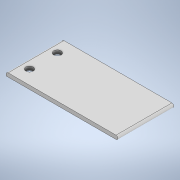
# Autodesk Inventor part: Cover
Saved by Autodesk Inventor 2020 (Build 240168000, 168)
## iProperties
Created: 2020-02-19
Part Number: Cover
Material: Generic
Document SubType Name: Modeling
Designer: maple
Density: 1 g/cm^3
Appearance: Default
Author: maple
Autodesk Inventor part; units mm, degrees
ref_plane "YZ Plane" through (0, 0, 0) normal (1, 0, 0) x (0, 1, 0)
ref_plane "XZ Plane" through (0, 0, 0) normal (0, 1, 0) x (-1, 0, 0)
ref_plane "XY Plane" through (0, 0, 0) normal (0, 0, 1) x (1, 0, 0)
sketch "Sketch1" plane through (0, 0, 0) normal (0, 1, 0) x (-1, 0, 0)
  line L0 (0, 0) -> (-76.2, 0)
  line L1 (-76.2, 0) -> (-76.2, -38.1)
  line L2 (-76.2, -38.1) -> (0, -38.1)
  line L3 (0, -38.1) -> (0, 0)
  dimension "d0" = 76.2
  dimension "d1" = 38.1
  constraints: 8 end point, 2 parallel, 1 horizontal, 1 perpendicular
  measures "d0" distance of L2.end L1.end
  measures "d1" distance of L1.end L0.end
extrude "Extrusion1" add sketch "Sketch1" along normal blind 2.54
sketch "Sketch2" plane through (0, 2.54, 0) normal (0, 1, 0) x (1, 0, 0)
  line L0 (0, 0) -> (6.35, 0)
  line L1 (0, 0) -> (76.2, 0) projected
  line L2 (6.35, 0) -> (6.35, 38.1)
  line L3 (76.2, 38.1) -> (0, 38.1) projected
  line L4 (6.35, 0) -> (6.35, 9.525)
  line L5 (6.35, 38.1) -> (6.35, 28.575)
  dimension "d4" = 6.35
  dimension "d5" = 9.525
  dimension "d6" = 9.525
  constraints: 8 end point, 4 point on line, 1 perpendicular
  measures "d4" distance of L0.start L0.end
  measures "d5" distance of L0.end L4.end
  measures "d6" distance of L2.end L5.end
hole "Hole1" at (6.35, 2.54, -9.525) at (6.35, 2.54, -28.575) direction (0, -1, 0) diameter 5.08 end through all
fillet "Fillet1" radius 1.27 2 edges at (76.2, 2.54, -19.05) (76.2, 0, -19.05)
fillet "Fillet2" radius 1.27 1 edges at (0, 2.54, -19.05)
body "Solid1"
